Autodesk Fusion 360 part; units mm, degrees
note: some values were not read from the file. Set by a fixed rule: which sketch regions a step uses.
(part 2 of 15)
  line L768 (243.501, -127.288) -> (243.645, -127.172)
  line L769 (233.618, -130.511) -> (233.477, -130.391)
  line L770 (245.044, -127.604) -> (245.097, -127.782)
  line L771 (245.116, -127.966) -> (245.115, -127.993)
  line L772 (244.675, -128.769) -> (244.509, -128.852)
  line L773 (243.482, -128.626) -> (243.367, -128.481)
  line L774 (101.127, -129.506) -> (101.145, -129.691)
  line L775 (244.509, -128.852) -> (244.331, -128.902)
  line L776 (99.2447, -129.677) -> (99.2654, -129.493)
  line L777 (99.8143, -130.561) -> (99.6524, -130.471)
  line L778 (100.201, -128.741) -> (100.386, -128.76)
  line L779 (233.982, -128.798) -> (234.167, -128.781)
  line L780 (99.6524, -130.471) -> (99.5112, -130.351)
  line L781 (244.357, -127.036) -> (244.534, -127.091)
  line L782 (99.6744, -128.896) -> (99.8387, -128.81)
  line L783 (245.097, -127.782) -> (245.116, -127.966)
  line L784 (243.382, -127.43) -> (243.501, -127.288)
  line L785 (100.36, -130.626) -> (100.175, -130.64)
  line L786 (243.236, -127.769) -> (243.292, -127.592)
  line L787 (243.292, -127.592) -> (243.382, -127.43)
  line L788 (244.172, -127.017) -> (244.357, -127.036)
  line L789 (99.4108, -129.154) -> (99.5299, -129.012)
  line L790 (244.942, -128.514) -> (244.821, -128.654)
  line L791 (245.092, -128.177) -> (245.033, -128.353)
  line L792 (99.3214, -129.316) -> (99.4108, -129.154)
  line L793 (245.115, -127.993) -> (245.092, -128.177)
  line L794 (99.5299, -129.012) -> (99.6744, -128.896)
  line L795 (243.81, -127.086) -> (243.988, -127.033)
  line L796 (243.988, -127.033) -> (244.172, -127.017)
  line L797 (233.225, -129.902) -> (233.21, -129.717)
  line L798 (244.84, -127.297) -> (244.957, -127.441)
  line L799 (100.017, -128.758) -> (100.201, -128.741)
  line L800 (99.8387, -128.81) -> (100.017, -128.758)
  line L801 (243.216, -127.953) -> (243.236, -127.769)
  line L802 (243.623, -128.747) -> (243.482, -128.626)
  line L803 (101.073, -129.329) -> (101.127, -129.506)
  line L804 (234.14, -130.681) -> (233.956, -130.659)
  line L805 (243.962, -128.894) -> (243.785, -128.837)
  line L806 (233.956, -130.659) -> (233.78, -130.601)
  line L807 (233.78, -130.601) -> (233.618, -130.511)
  line L808 (99.2654, -129.493) -> (99.3214, -129.316)
  line L809 (99.9906, -130.619) -> (99.8143, -130.561)
  line L810 (99.2602, -129.862) -> (99.2447, -129.677)
  line L811 (243.785, -128.837) -> (243.623, -128.747)
  line L812 (245.033, -128.353) -> (244.942, -128.514)
  line L813 (99.5112, -130.351) -> (99.3961, -130.205)
  line L814 (91.1154, -128.137) -> (91.0568, -128.313)
  line L815 (91.0568, -128.313) -> (90.9653, -128.474)
  line L816 (244.146, -128.916) -> (243.962, -128.894)
  line L817 (234.167, -128.781) -> (234.351, -128.8)
  line L818 (244.821, -128.654) -> (244.675, -128.769)
  line L819 (99.3961, -130.205) -> (99.3113, -130.04)
  line L820 (99.3113, -130.04) -> (99.2602, -129.862)
  line L821 (233.231, -129.533) -> (233.287, -129.357)
  line L822 (100.538, -130.576) -> (100.36, -130.626)
  line L823 (244.957, -127.441) -> (245.044, -127.604)
  line L824 (89.2391, -127.913) -> (89.2597, -127.729)
  line L825 (258.114, -121.378) -> (258.378, -121.48)
  line L826 (89.4051, -127.39) -> (89.5243, -127.248)
  line L827 (91.0673, -127.564) -> (91.1209, -127.742)
  line L828 (243.231, -128.138) -> (243.216, -127.953)
  line L829 (90.7202, -127.139) -> (90.8631, -127.257)
  line L830 (91.1209, -127.742) -> (91.139, -127.926)
  line L831 (258.378, -121.48) -> (258.624, -121.618)
  line L832 (90.698, -128.729) -> (90.5325, -128.812)
  line L833 (259.215, -122.218) -> (259.349, -122.466)
  line L834 (259.349, -122.466) -> (259.447, -122.731)
  line L835 (259.506, -123.008) -> (259.526, -123.289)
  line L836 (89.6468, -128.707) -> (89.5056, -128.586)
  line L837 (89.3158, -127.552) -> (89.4051, -127.39)
  line L838 (259.526, -123.289) -> (259.522, -123.415)
  line L839 (90.5325, -128.812) -> (90.3539, -128.862)
  line L840 (89.8331, -127.046) -> (90.011, -126.993)
  line L841 (90.8441, -128.614) -> (90.698, -128.729)
  line L842 (91.1386, -127.953) -> (91.1154, -128.137)
  line L843 (90.3539, -128.862) -> (90.1691, -128.876)
  line L844 (90.5571, -127.051) -> (90.7202, -127.139)
  line L845 (90.9802, -127.401) -> (91.0673, -127.564)
  line L846 (89.3904, -128.441) -> (89.3057, -128.276)
  line L847 (89.8086, -128.797) -> (89.6468, -128.707)
  line L848 (89.2597, -127.729) -> (89.3158, -127.552)
  line L849 (257.839, -121.314) -> (258.114, -121.378)
  line L850 (258.624, -121.618) -> (258.849, -121.789)
  line L851 (258.849, -121.789) -> (259.047, -121.99)
  line L852 (259.447, -122.731) -> (259.506, -123.008)
  line L853 (244.331, -128.902) -> (244.146, -128.916)
  line L854 (243.645, -127.172) -> (243.81, -127.086)
  line L855 (89.6688, -127.131) -> (89.8331, -127.046)
  line L856 (90.011, -126.993) -> (90.1956, -126.976)
  line L857 (90.1691, -128.876) -> (89.985, -128.854)
  line L858 (89.2546, -128.098) -> (89.2391, -127.913)
  line L859 (91.139, -127.926) -> (91.1386, -127.953)
  line L860 (90.38, -126.996) -> (90.5571, -127.051)
  line L861 (259.047, -121.99) -> (259.215, -122.218)
  line L862 (89.985, -128.854) -> (89.8086, -128.797)
  line L863 (90.1956, -126.976) -> (90.38, -126.996)
  line L864 (243.282, -128.316) -> (243.231, -128.138)
  line L865 (89.5056, -128.586) -> (89.3904, -128.441)
  line L866 (255.73, -122.409) -> (255.872, -122.165)
  line L867 (256.251, -121.748) -> (256.481, -121.584)
  line L868 (89.5243, -127.248) -> (89.6688, -127.131)
  line L869 (89.3057, -128.276) -> (89.2546, -128.098)
  line L870 (90.8631, -127.257) -> (90.9802, -127.401)
  line L871 (90.9653, -128.474) -> (90.8441, -128.614)
  line L872 (257.993, -125.234) -> (257.715, -125.28)
  line L873 (257.715, -125.28) -> (257.432, -125.287)
  line L874 (255.538, -123.509) -> (255.527, -123.227)
  line L875 (56.6309, -103.238) -> (56.4848, -103.352)
  line L876 (298.503, -101.671) -> (298.556, -101.849)
  line L877 (55.4336, -103.33) -> (55.2924, -103.21)
  line L878 (55.5955, -103.42) -> (55.4336, -103.33)
  line L879 (55.0466, -102.352) -> (55.1026, -102.176)
  line L880 (55.3111, -101.871) -> (55.4556, -101.755)
  line L881 (298.556, -101.849) -> (298.574, -102.033)
  line L882 (298.416, -101.508) -> (298.503, -101.671)
  line L883 (298.299, -101.364) -> (298.416, -101.508)
  line L884 (298.551, -102.244) -> (298.492, -102.42)
  line L885 (55.9559, -103.5) -> (55.7718, -103.478)
  line L886 (55.1026, -102.176) -> (55.1919, -102.013)
  line L887 (55.0925, -102.9) -> (55.0414, -102.721)
  line L888 (55.7978, -101.617) -> (55.9824, -101.6)
  line L889 (298.574, -102.06) -> (298.551, -102.244)
  line L890 (56.4848, -103.352) -> (56.3193, -103.436)
  line L891 (55.2924, -103.21) -> (55.1773, -103.064)
  line L892 (55.9824, -101.6) -> (56.1668, -101.619)
  line L893 (55.0414, -102.721) -> (55.0259, -102.537)
  line L894 (297.993, -101.158) -> (298.156, -101.246)
  line L895 (55.4556, -101.755) -> (55.6199, -101.669)
  line L896 (297.815, -101.103) -> (297.993, -101.158)
  line L897 (298.574, -102.033) -> (298.574, -102.06)
  line L898 (55.0259, -102.537) -> (55.0466, -102.352)
  line L899 (55.1919, -102.013) -> (55.3111, -101.871)
  line L900 (59.8286, -105.068) -> (59.6095, -104.89)
  line L901 (269.323, -104.381) -> (269.299, -104.565)
  line L902 (269.149, -104.902) -> (269.028, -105.042)
  line L903 (269.028, -105.042) -> (268.882, -105.156)
  line L904 (59.0765, -102.814) -> (59.1826, -102.552)
  line L905 (268.904, -103.567) -> (269.047, -103.685)
  line L906 (268.564, -103.424) -> (268.741, -103.478)
  line L907 (58.9796, -103.369) -> (59.0084, -103.088)
  line L908 (66.9311, -104.341) -> (66.9078, -104.525)
  line L909 (66.9078, -104.525) -> (66.8493, -104.7)
  line L910 (267.49, -104.704) -> (267.439, -104.526)
  line L911 (267.5, -103.98) -> (267.589, -103.817)
  line L912 (268.195, -103.421) -> (268.38, -103.404)
  line L913 (66.3496, -103.438) -> (66.5127, -103.527)
  line L914 (268.017, -103.473) -> (268.195, -103.421)
  line L915 (267.831, -105.134) -> (267.69, -105.014)
  line L916 (65.1829, -104.829) -> (65.0981, -104.664)
  line L917 (294.542, -102.358) -> (294.602, -102.634)
  line L918 (65.1083, -103.94) -> (65.1976, -103.777)
  line L919 (66.9133, -104.13) -> (66.9314, -104.314)
  line L920 (65.7774, -105.242) -> (65.6011, -105.185)
  line L921 (66.7727, -103.788) -> (66.8598, -103.952)
  line L922 (59.7038, -101.891) -> (59.9336, -101.727)
  line L923 (66.9314, -104.314) -> (66.9311, -104.341)
  line L924 (66.8493, -104.7) -> (66.7577, -104.862)
  line L925 (66.6555, -103.645) -> (66.7727, -103.788)
  line L926 (268.538, -105.29) -> (268.353, -105.304)
  line L927 (267.423, -104.341) -> (267.444, -104.157)
  line L928 (59.4994, -102.086) -> (59.7038, -101.891)
  line L929 (267.993, -105.225) -> (267.831, -105.134)
  line L930 (267.589, -103.817) -> (267.708, -103.675)
  line L931 (268.353, -105.304) -> (268.169, -105.282)
  line L932 (66.8598, -103.952) -> (66.9133, -104.13)
  line L933 (66.7577, -104.862) -> (66.6366, -105.002)
  line L934 (267.575, -104.869) -> (267.49, -104.704)
  line L935 (267.439, -104.526) -> (267.423, -104.341)
  line L936 (268.169, -105.282) -> (267.993, -105.225)
  line L937 (267.853, -103.559) -> (268.017, -103.473)
  line L938 (66.1725, -103.384) -> (66.3496, -103.438)
  line L939 (267.444, -104.157) -> (267.5, -103.98)
  line L940 (267.708, -103.675) -> (267.853, -103.559)
  line L941 (268.882, -105.156) -> (268.717, -105.24)
  line L942 (268.38, -103.404) -> (268.564, -103.424)
  line L943 (66.5127, -103.527) -> (66.6555, -103.645)
  line L944 (268.717, -105.24) -> (268.538, -105.29)
  line L945 (267.69, -105.014) -> (267.575, -104.869)
  line L946 (269.251, -103.992) -> (269.305, -104.17)
  line L947 (60.7279, -101.448) -> (61.01, -101.432)
  line L948 (60.1843, -101.596) -> (60.4509, -101.503)
  line L949 (269.241, -104.741) -> (269.149, -104.902)
  line L950 (59.0084, -103.088) -> (59.0765, -102.814)
  line L951 (59.9336, -101.727) -> (60.1843, -101.596)
  line L952 (269.299, -104.565) -> (269.241, -104.741)
  line L953 (269.323, -104.354) -> (269.323, -104.381)
  line L954 (61.01, -101.432) -> (61.2915, -101.457)
  line L955 (59.2571, -104.45) -> (59.1309, -104.197)
  line L956 (269.305, -104.17) -> (269.323, -104.354)
  line L957 (269.164, -103.828) -> (269.251, -103.992)
  line L958 (59.0414, -103.929) -> (58.9907, -103.651)
  line L959 (60.4509, -101.503) -> (60.7279, -101.448)
  line L960 (268.741, -103.478) -> (268.904, -103.567)
  line L961 (269.047, -103.685) -> (269.164, -103.828)
  line L962 (59.4178, -104.682) -> (59.2571, -104.45)
  line L963 (59.3245, -102.308) -> (59.4994, -102.086)
  line L964 (59.1826, -102.552) -> (59.3245, -102.308)
  line L965 (59.6095, -104.89) -> (59.4178, -104.682)
  line L966 (109.335, -72.8722) -> (109.454, -72.7302)
  line L967 (278.888, -103.392) -> (278.722, -103.476)
  line L968 (56.3439, -101.674) -> (56.507, -101.762)
  line L969 (278.359, -103.54) -> (278.175, -103.518)
  line L970 (55.1773, -103.064) -> (55.0925, -102.9)
  line L971 (277.495, -102.94) -> (277.444, -102.761)
  line L972 (278.201, -101.657) -> (278.385, -101.64)
  line L973 (277.444, -102.761) -> (277.429, -102.577)
  line L974 (278.175, -103.518) -> (277.998, -103.46)
  line L975 (278.385, -101.64) -> (278.57, -101.659)
  line L976 (278.722, -103.476) -> (278.544, -103.525)
  line L977 (298.156, -101.246) -> (298.299, -101.364)
  line L978 (56.3193, -103.436) -> (56.1408, -103.485)
  line L979 (74.2602, -103.232) -> (74.3495, -103.07)
  line L980 (279.053, -101.92) -> (279.17, -102.064)
  line L981 (279.155, -103.138) -> (279.034, -103.278)
  line L982 (74.753, -104.477) -> (74.5912, -104.387)
  line L983 (56.9077, -102.365) -> (56.9258, -102.55)
  line L984 (277.859, -101.795) -> (278.023, -101.709)
  line L985 (277.695, -103.25) -> (277.58, -103.105)
  line L986 (277.429, -102.577) -> (277.449, -102.392)
  line L987 (277.714, -101.911) -> (277.859, -101.795)
  line L988 (56.1668, -101.619) -> (56.3439, -101.674)
  line L989 (277.595, -102.053) -> (277.714, -101.911)
  line L990 (74.3495, -103.07) -> (74.4687, -102.928)
  line L991 (74.1989, -103.778) -> (74.1834, -103.593)
  line L992 (277.506, -102.216) -> (277.595, -102.053)
  line L993 (74.2501, -103.956) -> (74.1989, -103.778)
  line L994 (279.257, -102.228) -> (279.311, -102.405)
  line L995 (56.7671, -102.024) -> (56.8541, -102.188)
  line L996 (277.449, -102.392) -> (277.506, -102.216)
  line L997 (279.328, -102.616) -> (279.305, -102.8)
  line L998 (279.329, -102.59) -> (279.328, -102.616)
  line L999 (74.9293, -104.534) -> (74.753, -104.477)
  line L1000 (279.034, -103.278) -> (278.888, -103.392)
  line L1001 (56.9254, -102.576) -> (56.9022, -102.76)
  line L1002 (56.6499, -101.88) -> (56.7671, -102.024)
  line L1003 (56.9022, -102.76) -> (56.8437, -102.936)
  line L1004 (279.305, -102.8) -> (279.247, -102.976)
  line L1005 (56.9258, -102.55) -> (56.9254, -102.576)
  line L1006 (278.57, -101.659) -> (278.747, -101.714)
  line L1007 (56.8437, -102.936) -> (56.7521, -103.097)
  line L1008 (56.7521, -103.097) -> (56.6309, -103.238)
  line L1009 (56.8541, -102.188) -> (56.9077, -102.365)
  line L1010 (278.023, -101.709) -> (278.201, -101.657)
  line L1011 (277.998, -103.46) -> (277.837, -103.37)
  line L1012 (278.544, -103.525) -> (278.359, -103.54)
  line L1013 (56.507, -101.762) -> (56.6499, -101.88)
  line L1014 (277.837, -103.37) -> (277.695, -103.25)
  line L1015 (75.4769, -104.492) -> (75.2983, -104.542)
  line L1016 (277.58, -103.105) -> (277.495, -102.94)
  line L1017 (74.2041, -103.409) -> (74.2602, -103.232)
  line L1018 (74.4687, -102.928) -> (74.6132, -102.812)
  line L1019 (279.247, -102.976) -> (279.155, -103.138)
  line L1020 (278.747, -101.714) -> (278.91, -101.802)
  line L1021 (74.45, -104.266) -> (74.3348, -104.121)
  line L1022 (30.5232, -111.407) -> (30.7847, -111.468)
  line L1023 (112.793, -114.541) -> (112.811, -114.725)
  line L1024 (112.652, -114.199) -> (112.739, -114.363)
  line L1025 (112.516, -115.413) -> (112.37, -115.527)
  line L1026 (111.318, -115.505) -> (111.177, -115.385)
  line L1027 (112.204, -115.611) -> (112.026, -115.661)
  line L1028 (111.177, -115.385) -> (111.062, -115.24)
  line L1029 (112.787, -114.936) -> (112.728, -115.111)
  line L1030 (111.062, -115.24) -> (110.977, -115.075)
  line L1031 (111.34, -113.93) -> (111.505, -113.844)
  line L1032 (112.637, -115.273) -> (112.516, -115.413)
  line L1033 (111.841, -115.675) -> (111.657, -115.653)
  line L1034 (111.196, -114.046) -> (111.34, -113.93)
  line L1035 (32.0506, -112.754) -> (32.107, -113.016)
  line L1036 (28.9254, -114.669) -> (28.7432, -114.472)
  line L1037 (29.6106, -115.082) -> (29.3634, -114.977)
  line L1038 (31.4825, -111.859) -> (31.6708, -112.05)
  line L1039 (111.077, -114.188) -> (111.196, -114.046)
  line L1040 (31.9052, -114.173) -> (31.7631, -114.401)
  line L1041 (31.5904, -114.606) -> (31.3905, -114.785)
  line L1042 (32.0137, -113.928) -> (31.9052, -114.173)
  line L1043 (31.7631, -114.401) -> (31.5904, -114.606)
  line L1044 (31.1674, -114.934) -> (30.9254, -115.051)
  line L1045 (31.2691, -111.696) -> (31.4825, -111.859)
  line L1046 (29.3634, -114.977) -> (29.1335, -114.838)
  line L1047 (30.1365, -115.182) -> (29.87, -115.15)
  line L1048 (28.3857, -113.757) -> (28.3375, -113.492)
  line L1049 (31.3905, -114.785) -> (31.1674, -114.934)
  line L1050 (28.4706, -114.011) -> (28.3857, -113.757)
  line L1051 (31.9577, -112.502) -> (32.0506, -112.754)
  line L1052 (30.7847, -111.468) -> (31.035, -111.565)
  line L1053 (31.035, -111.565) -> (31.2691, -111.696)
  line L1054 (30.4048, -115.176) -> (30.1365, -115.182)
  line L1055 (29.87, -115.15) -> (29.6106, -115.082)
  line L1056 (31.6708, -112.05) -> (31.8302, -112.266)
  line L1057 (28.5906, -114.251) -> (28.4706, -114.011)
  line L1058 (30.9254, -115.051) -> (30.6695, -115.132)
  line L1059 (28.3375, -113.492) -> (28.3269, -113.224)
  line L1060 (32.107, -113.016) -> (32.126, -113.284)
  line L1061 (31.8302, -112.266) -> (31.9577, -112.502)
  line L1062 (30.6695, -115.132) -> (30.4048, -115.176)
  line L1063 (32.126, -113.284) -> (32.1223, -113.403)
  line L1064 (28.7432, -114.472) -> (28.5906, -114.251)
  line L1065 (116.489, -117.572) -> (116.216, -117.499)
  line L1066 (114.893, -115.263) -> (114.961, -114.989)
  line L1067 (115.209, -114.483) -> (115.384, -114.261)
  line L1068 (116.216, -117.499) -> (115.955, -117.389)
  line L1069 (114.864, -115.544) -> (114.893, -115.263)
  line L1070 (212.856, -115.654) -> (213.019, -115.742)
  line L1071 (211.554, -116.701) -> (211.538, -116.516)
  line L1072 (213.438, -116.556) -> (213.415, -116.74)
  line L1073 (116.895, -113.607) -> (117.176, -113.632)
  line L1074 (212.679, -115.599) -> (212.856, -115.654)
  line L1075 (117.6, -117.467) -> (117.33, -117.552)
  line L1076 (117.33, -117.552) -> (117.052, -117.598)
  line L1077 (115.142, -116.625) -> (115.016, -116.373)
  line L1078 (213.438, -116.529) -> (213.438, -116.556)
  line L1079 (211.538, -116.516) -> (211.559, -116.332)
  line L1080 (122.234, -115.614) -> (122.397, -115.702)
  line L1081 (116.613, -113.623) -> (116.895, -113.607)
  line L1082 (115.384, -114.261) -> (115.589, -114.066)
  line L1083 (122.397, -115.702) -> (122.54, -115.82)
  line L1084 (114.961, -114.989) -> (115.067, -114.727)
  line L1085 (211.704, -115.993) -> (211.824, -115.851)
  line L1086 (215.695, -114.767) -> (215.837, -114.523)
  line L1087 (115.713, -117.244) -> (115.494, -117.065)
  line L1088 (213.143, -117.217) -> (212.997, -117.332)
  line L1089 (122.057, -115.559) -> (122.234, -115.614)
  line L1090 (213.42, -116.345) -> (213.438, -116.529)
  line L1091 (117.052, -117.598) -> (116.769, -117.605)
  line L1092 (122.54, -115.82) -> (122.658, -115.964)
  line L1093 (213.367, -116.167) -> (213.42, -116.345)
  line L1094 (213.28, -116.004) -> (213.367, -116.167)
  line L1095 (213.415, -116.74) -> (213.356, -116.916)
  line L1096 (215.837, -114.523) -> (216.012, -114.301)
  line L1097 (115.589, -114.066) -> (115.818, -113.902)
  line L1098 (116.336, -113.678) -> (116.613, -113.623)
  line L1099 (115.303, -116.858) -> (115.142, -116.625)
  line L1100 (211.824, -115.851) -> (211.968, -115.735)
  line L1101 (212.132, -115.649) -> (212.31, -115.596)
  line L1102 (115.818, -113.902) -> (116.069, -113.772)
  line L1103 (216.446, -113.942) -> (216.697, -113.812)
  line L1104 (116.069, -113.772) -> (116.336, -113.678)
  line L1105 (115.494, -117.065) -> (115.303, -116.858)
  line L1106 (212.997, -117.332) -> (212.832, -117.415)
  line L1107 (114.875, -115.827) -> (114.864, -115.544)
  line L1108 (213.265, -117.077) -> (213.143, -117.217)
  line L1109 (215.492, -115.584) -> (215.521, -115.303)
  line L1110 (115.955, -117.389) -> (115.713, -117.244)
  line L1111 (114.926, -116.105) -> (114.875, -115.827)
  line L1112 (213.162, -115.86) -> (213.28, -116.004)
  line L1113 (212.495, -115.579) -> (212.679, -115.599)
  line L1114 (115.067, -114.727) -> (115.209, -114.483)
  line L1115 (213.019, -115.742) -> (213.162, -115.86)
  line L1116 (115.016, -116.373) -> (114.926, -116.105)
  line L1117 (116.769, -117.605) -> (116.489, -117.572)
  line L1118 (-10.9606, -114.234) -> (-10.7834, -114.289)
  line L1119 (122.521, -117.177) -> (122.375, -117.291)
  line L1120 (121.846, -117.439) -> (121.662, -117.417)
  line L1121 (122.031, -117.425) -> (121.846, -117.439)
  line L1122 (211.946, -117.31) -> (211.805, -117.189)
  line L1123 (211.559, -116.332) -> (211.615, -116.155)
  line L1124 (-10.2197, -114.98) -> (-10.2016, -115.165)
  line L1125 (212.284, -117.457) -> (212.108, -117.4)
  line L1126 (-10.9866, -116.1) -> (-11.1715, -116.114)
  line L1127 (121.486, -117.36) -> (121.324, -117.269)
  line L1128 (122.745, -116.127) -> (122.798, -116.305)
  line L1129 (-11.8163, -114.486) -> (-11.6718, -114.37)
  line L1130 (122.793, -116.7) -> (122.734, -116.876)
  line L1131 (-11.1449, -114.215) -> (-10.9606, -114.234)
  line L1132 (-12.1015, -115.151) -> (-12.0808, -114.967)
  line L1133 (222.685, -113.835) -> (222.862, -113.889)
  line L1134 (-10.808, -116.05) -> (-10.9866, -116.1)
  line L1135 (121.082, -115.953) -> (121.202, -115.811)
  line L1136 (-10.6425, -115.967) -> (-10.808, -116.05)
  line L1137 (212.653, -117.465) -> (212.468, -117.479)
  line L1138 (-10.7834, -114.289) -> (-10.6203, -114.377)
  line L1139 (121.873, -115.539) -> (122.057, -115.559)
  line L1140 (-10.4775, -114.495) -> (-10.3603, -114.639)
  line L1141 (121.346, -115.694) -> (121.51, -115.609)
  line L1142 (121.51, -115.609) -> (121.688, -115.556)
  line L1143 (122.375, -117.291) -> (122.21, -117.375)
  line L1144 (121.688, -115.556) -> (121.873, -115.539)
  line L1145 (-10.3753, -115.712) -> (-10.4964, -115.853)
  line L1146 (211.605, -116.879) -> (211.554, -116.701)
  line L1147 (212.468, -117.479) -> (212.284, -117.457)
  line L1148 (212.31, -115.596) -> (212.495, -115.579)
  line L1149 (121.662, -117.417) -> (121.486, -117.36)
  line L1150 (120.983, -116.839) -> (120.932, -116.661)
  line L1151 (-11.6718, -114.37) -> (-11.5075, -114.284)
  line L1152 (-12.086, -115.336) -> (-12.1015, -115.151)
  line L1153 (-11.3296, -114.231) -> (-11.1449, -114.215)
  line L1154 (-11.5075, -114.284) -> (-11.3296, -114.231)
  line L1155 (212.108, -117.4) -> (211.946, -117.31)
  line L1156 (212.832, -117.415) -> (212.653, -117.465)
  line L1157 (211.805, -117.189) -> (211.69, -117.044)
  line L1158 (122.21, -117.375) -> (122.031, -117.425)
  line L1159 (122.798, -116.305) -> (122.816, -116.489)
  line L1160 (120.916, -116.476) -> (120.937, -116.292)
  line L1161 (-10.2837, -115.551) -> (-10.3753, -115.712)
  line L1162 (-11.1715, -116.114) -> (-11.3556, -116.092)
  line L1163 (121.183, -117.149) -> (121.068, -117.004)
  line L1164 (121.068, -117.004) -> (120.983, -116.839)
  line L1165 (122.816, -116.489) -> (122.816, -116.516)
  line L1166 (-10.6203, -114.377) -> (-10.4775, -114.495)
  line L1167 (121.202, -115.811) -> (121.346, -115.694)
  line L1168 (122.816, -116.516) -> (122.793, -116.7)
  line L1169 (121.324, -117.269) -> (121.183, -117.149)
  line L1170 (120.932, -116.661) -> (120.916, -116.476)
  line L1171 (211.69, -117.044) -> (211.605, -116.879)
  line L1172 (120.937, -116.292) -> (120.993, -116.115)
  line L1173 (122.643, -117.037) -> (122.521, -117.177)
  line L1174 (-10.2016, -115.165) -> (-10.2019, -115.191)
  line L1175 (-10.2019, -115.191) -> (-10.2252, -115.375)
  line L1176 (122.658, -115.964) -> (122.745, -116.127)
  line L1177 (213.356, -116.916) -> (213.265, -117.077)
  line L1178 (122.734, -116.876) -> (122.643, -117.037)
  line L1179 (120.993, -116.115) -> (121.082, -115.953)
  line L1180 (211.615, -116.155) -> (211.704, -115.993)
  line L1181 (211.968, -115.735) -> (212.132, -115.649)
  line L1182 (221.695, -115.28) -> (221.611, -115.115)
  line L1183 (-10.2252, -115.375) -> (-10.2837, -115.551)
  line L1184 (222.316, -113.832) -> (222.501, -113.815)
  line L1185 (-12.0808, -114.967) -> (-12.0248, -114.79)
  line L1186 (223.444, -114.765) -> (223.444, -114.792)
  line L1187 (222.29, -115.693) -> (222.114, -115.636)
  line L1188 (223.362, -115.152) -> (223.27, -115.313)
  line L1189 (222.474, -115.715) -> (222.29, -115.693)
  line L1190 (222.501, -113.815) -> (222.685, -113.835)
  line L1191 (221.544, -114.752) -> (221.565, -114.568)
  line L1192 (-11.835, -115.824) -> (-11.9501, -115.679)
  line L1193 (223.285, -114.239) -> (223.372, -114.403)
  line L1194 (-10.3603, -114.639) -> (-10.2733, -114.803)
  line L1195 (223.025, -113.978) -> (223.168, -114.096)
  line L1196 (112.026, -115.661) -> (111.841, -115.675)
  line L1197 (-12.0248, -114.79) -> (-11.9354, -114.628)
  line L1198 (223.149, -115.453) -> (223.003, -115.567)
  line L1199 (112.052, -113.795) -> (112.229, -113.849)
  line L1200 (223.42, -114.976) -> (223.362, -115.152)
  line L1201 (111.48, -115.596) -> (111.318, -115.505)
  line L1202 (222.138, -113.884) -> (222.316, -113.832)
  line L1203 (223.444, -114.792) -> (223.42, -114.976)
  line L1204 (110.911, -114.712) -> (110.931, -114.528)
  line L1205 (221.829, -114.086) -> (221.974, -113.97)
  line L1206 (112.37, -115.527) -> (112.204, -115.611)
  line L1207 (112.535, -114.056) -> (112.652, -114.199)
  line L1208 (221.621, -114.391) -> (221.71, -114.228)
  line L1209 (112.739, -114.363) -> (112.793, -114.541)
  line L1210 (-11.9501, -115.679) -> (-12.0349, -115.514)
  line L1211 (221.974, -113.97) -> (222.138, -113.884)
  line L1212 (112.229, -113.849) -> (112.392, -113.938)
  line L1213 (221.952, -115.545) -> (221.811, -115.425)
  line L1214 (223.27, -115.313) -> (223.149, -115.453)
  line L1215 (222.659, -115.701) -> (222.474, -115.715)
  line L1216 (112.392, -113.938) -> (112.535, -114.056)
  line L1217 (111.657, -115.653) -> (111.48, -115.596)
  line L1218 (223.003, -115.567) -> (222.837, -115.651)
  line L1219 (223.168, -114.096) -> (223.285, -114.239)
  line L1220 (112.81, -114.752) -> (112.787, -114.936)
  line L1221 (222.837, -115.651) -> (222.659, -115.701)
  line L1222 (-11.3556, -116.092) -> (-11.5319, -116.035)
  line L1223 (223.372, -114.403) -> (223.426, -114.581)
  line L1224 (221.565, -114.568) -> (221.621, -114.391)
  line L1225 (112.728, -115.111) -> (112.637, -115.273)
  line L1226 (111.683, -113.792) -> (111.867, -113.775)
  line L1227 (221.71, -114.228) -> (221.829, -114.086)
  line L1228 (-10.2733, -114.803) -> (-10.2197, -114.98)
  line L1229 (221.611, -115.115) -> (221.56, -114.937)
  line L1230 (221.56, -114.937) -> (221.544, -114.752)
  line L1231 (112.811, -114.725) -> (112.81, -114.752)
  line L1232 (110.977, -115.075) -> (110.926, -114.897)
  line L1233 (110.926, -114.897) -> (110.911, -114.712)
  line L1234 (110.987, -114.351) -> (111.077, -114.188)
  line L1235 (111.505, -113.844) -> (111.683, -113.792)
  line L1236 (-11.6938, -115.945) -> (-11.835, -115.824)
  line L1237 (-12.0349, -115.514) -> (-12.086, -115.336)
  line L1238 (110.931, -114.528) -> (110.987, -114.351)
  line L1239 (222.114, -115.636) -> (221.952, -115.545)
  line L1240 (-11.9354, -114.628) -> (-11.8163, -114.486)
  line L1241 (-11.5319, -116.035) -> (-11.6938, -115.945)
  line L1242 (223.426, -114.581) -> (223.444, -114.765)
  line L1243 (221.811, -115.425) -> (221.695, -115.28)
  line L1244 (222.862, -113.889) -> (223.025, -113.978)
  line L1245 (-10.4964, -115.853) -> (-10.6425, -115.967)
  line L1246 (111.867, -113.775) -> (112.052, -113.795)
  line L1247 (294.31, -101.844) -> (294.444, -102.093)
  line L1248 (65.0522, -104.117) -> (65.1083, -103.94)
  line L1249 (65.0981, -104.664) -> (65.047, -104.486)
  line L1250 (294.602, -102.634) -> (294.622, -102.916)
  line L1251 (65.8034, -103.381) -> (65.9881, -103.364)
  line L1252 (293.944, -101.415) -> (294.142, -101.617)
  line L1253 (65.9615, -105.264) -> (65.7774, -105.242)
  line L1254 (66.6366, -105.002) -> (66.4905, -105.116)
  line L1255 (65.0315, -104.301) -> (65.0522, -104.117)
  line L1256 (293.473, -101.106) -> (293.72, -101.244)
  line L1257 (65.2981, -104.974) -> (65.1829, -104.829)
  line L1258 (66.1464, -105.25) -> (65.9615, -105.264)
  line L1259 (66.325, -105.2) -> (66.1464, -105.25)
  line L1260 (294.142, -101.617) -> (294.31, -101.844)
  line L1261 (294.444, -102.093) -> (294.542, -102.358)
  line L1262 (290.684, -103.413) -> (290.634, -103.135)
  line L1263 (290.9, -103.934) -> (290.774, -103.681)
  line L1264 (294.618, -103.041) -> (294.58, -103.321)
  line L1265 (294.24, -104.091) -> (294.058, -104.307)
  line L1266 (291.347, -101.375) -> (291.577, -101.21)
  line L1267 (290.967, -101.791) -> (291.142, -101.57)
  line L1268 (293.089, -104.86) -> (292.81, -104.907)
  line L1269 (291.061, -104.166) -> (290.9, -103.934)
  line L1270 (294.58, -103.321) -> (294.503, -103.593)
  line L1271 (291.827, -101.08) -> (292.094, -100.986)
  line L1272 (294.058, -104.307) -> (293.847, -104.496)
  line L1273 (291.253, -104.374) -> (291.061, -104.166)
  line L1274 (292.81, -104.907) -> (292.527, -104.913)
  line L1275 (291.142, -101.57) -> (291.347, -101.375)
  line L1276 (291.974, -104.808) -> (291.714, -104.698)
  line L1277 (290.623, -102.853) -> (290.651, -102.572)
  line L1278 (293.613, -104.653) -> (293.358, -104.775)
  line L1279 (290.774, -103.681) -> (290.684, -103.413)
  line L1280 (291.472, -104.552) -> (291.253, -104.374)
  line L1281 (290.826, -102.036) -> (290.967, -101.791)
  line L1282 (290.72, -102.298) -> (290.826, -102.036)
  line L1283 (292.094, -100.986) -> (292.371, -100.931)
  line L1284 (293.847, -104.496) -> (293.613, -104.653)
  line L1285 (294.389, -103.851) -> (294.24, -104.091)
  line L1286 (291.714, -104.698) -> (291.472, -104.552)
  line L1287 (291.577, -101.21) -> (291.827, -101.08)
  line L1288 (292.527, -104.913) -> (292.247, -104.88)
  line L1289 (290.634, -103.135) -> (290.623, -102.853)
  line L1290 (292.247, -104.88) -> (291.974, -104.808)
  line L1291 (294.503, -103.593) -> (294.389, -103.851)
  line L1292 (290.651, -102.572) -> (290.72, -102.298)
  line L1293 (293.358, -104.775) -> (293.089, -104.86)
  line L1294 (294.622, -102.916) -> (294.618, -103.041)
  line L1295 (293.21, -101.004) -> (293.473, -101.106)
  line L1296 (66.4905, -105.116) -> (66.325, -105.2)
  line L1297 (293.72, -101.244) -> (293.944, -101.415)
  line L1298 (65.9881, -103.364) -> (66.1725, -103.384)
  line L1299 (65.3168, -103.635) -> (65.4613, -103.519)
  line L1300 (65.047, -104.486) -> (65.0315, -104.301)
  line L1301 (65.1976, -103.777) -> (65.3168, -103.635)
  line L1302 (65.4393, -105.094) -> (65.2981, -104.974)
  line L1303 (65.6011, -105.185) -> (65.4393, -105.094)
  line L1304 (65.4613, -103.519) -> (65.6256, -103.433)
  line L1305 (65.6256, -103.433) -> (65.8034, -103.381)
  line L1306 (292.935, -100.94) -> (293.21, -101.004)
  line L1307 (17.0862, -99.0351) -> (17.035, -98.8569)
  line L1308 (-1.9892, -95.4764) -> (-1.7427, -95.6145)
  line L1309 (-4.6368, -96.4062) -> (-4.4949, -96.1619)
  line L1310 (-0.8447, -97.4117) -> (-0.8823, -97.6917)
  line L1311 (17.2861, -99.3453) -> (17.1709, -99.2)
  line L1312 (17.0963, -98.3111) -> (17.1856, -98.1487)
  line L1313 (18.8958, -98.8959) -> (18.8373, -99.0718)
  line L1314 (17.0195, -98.6721) -> (17.0402, -98.4879)
  line L1315 (17.035, -98.8569) -> (17.0195, -98.6721)
  line L1316 (17.6136, -97.8046) -> (17.7914, -97.7522)
  line L1317 (-4.7429, -96.668) -> (-4.6368, -96.4062)
  line L1318 (17.3048, -98.0066) -> (17.4493, -97.8905)
  line L1319 (-1.8498, -99.0233) -> (-2.1045, -99.1456)
  line L1320 (18.4785, -99.4875) -> (18.313, -99.5711)
  line L1321 (-4.2099, -98.744) -> (-4.4016, -98.5366)
  line L1322 (-4.8287, -97.5056) -> (-4.8398, -97.2233)
  line L1323 (17.9495, -99.6352) -> (17.7654, -99.6132)
  line L1324 (17.1709, -99.2) -> (17.0862, -99.0351)
  line L1325 (-4.6885, -98.0515) -> (-4.7779, -97.7835)
  line L1326 (-0.9202, -96.7281) -> (-0.8607, -97.0043)
  line L1327 (-2.5279, -95.3107) -> (-2.2527, -95.3745)
  line L1328 (-2.2527, -95.3745) -> (-1.9892, -95.4764)
  line L1329 (18.8373, -99.0718) -> (18.7457, -99.233)
  line L1330 (-1.3199, -95.9872) -> (-1.1521, -96.2144)
  line L1331 (17.5891, -99.5559) -> (17.4273, -99.4655)
  line L1332 (17.1856, -98.1487) -> (17.3048, -98.0066)
  line L1333 (17.7914, -97.7522) -> (17.9761, -97.7354)
  line L1334 (18.6246, -99.3734) -> (18.4785, -99.4875)
  line L1335 (17.7654, -99.6132) -> (17.5891, -99.5559)
  line L1336 (18.9194, -98.6854) -> (18.9191, -98.7119)
  line L1337 (17.9761, -97.7354) -> (18.1605, -97.7548)
  line L1338 (17.4493, -97.8905) -> (17.6136, -97.8046)
  line L1339 (-1.5181, -95.7859) -> (-1.3199, -95.9872)
  line L1340 (18.7457, -99.233) -> (18.6246, -99.3734)
  line L1341 (17.4273, -99.4655) -> (17.2861, -99.3453)
  line L1342 (18.9191, -98.7119) -> (18.8958, -98.8959)
  line L1343 (-4.5622, -98.3042) -> (-4.6885, -98.0515)
  line L1344 (18.1344, -99.621) -> (17.9495, -99.6352)
  line L1345 (-3.9908, -98.9224) -> (-4.2099, -98.744)
  line L1346 (17.0402, -98.4879) -> (17.0963, -98.3111)
  line L1347 (18.313, -99.5711) -> (18.1344, -99.621)
  line L1348 (-3.3685, -95.357) -> (-3.0914, -95.3019)
  line L1349 (-4.8398, -97.2233) -> (-4.811, -96.9422)
  line L1350 (3.0404, -97.8062) -> (3.094, -97.9837)
  line L1351 (2.1422, -99.118) -> (1.9581, -99.0961)
  line L1352 (1.7817, -99.0388) -> (1.6199, -98.9483)
  line L1353 (-3.2155, -99.2507) -> (-3.4886, -99.1783)
  line L1354 (3.1121, -98.1682) -> (3.1117, -98.1947)
  line L1355 (-0.8408, -97.2861) -> (-0.8447, -97.4117)
  line L1356 (-2.6525, -99.2772) -> (-2.935, -99.2839)
  line L1357 (1.6199, -98.9483) -> (1.4787, -98.8281)
  line L1358 (-1.6149, -98.8664) -> (-1.8498, -99.0233)
  line L1359 (2.6933, -97.3806) -> (2.8362, -97.4988)
  line L1360 (1.2122, -98.155) -> (1.2328, -97.9707)
  line L1361 (-1.1521, -96.2144) -> (-1.0179, -96.4631)
  line L1362 (2.6711, -98.9703) -> (2.5056, -99.0539)
  line L1363 (-4.32, -95.9401) -> (-4.1156, -95.7451)
  line L1364 (-3.4886, -99.1783) -> (-3.7487, -99.0681)
  line L1365 (-4.1156, -95.7451) -> (-3.8857, -95.5808)
  line L1366 (2.3531, -97.2376) -> (2.5302, -97.2924)
  line L1367 (2.5056, -99.0539) -> (2.327, -99.1038)
  line L1368 (-2.935, -99.2839) -> (-3.2155, -99.2507)
  line L1369 (2.9384, -98.7158) -> (2.8172, -98.8562)
  line L1370 (2.8172, -98.8562) -> (2.6711, -98.9703)
  line L1371 (-3.8857, -95.5808) -> (-3.6351, -95.4506)
  line L1372 (3.1117, -98.1947) -> (3.0885, -98.3787)
  line L1373 (-1.4045, -98.6779) -> (-1.6149, -98.8664)
  line L1374 (-4.811, -96.9422) -> (-4.7429, -96.668)
  line L1375 (-1.2227, -98.4617) -> (-1.4045, -98.6779)
  line L1376 (-3.6351, -95.4506) -> (-3.3685, -95.357)
  line L1377 (1.3635, -98.6828) -> (1.2788, -98.5179)
  line L1378 (-2.8093, -95.2863) -> (-2.5279, -95.3107)
  line L1379 (2.8362, -97.4988) -> (2.9533, -97.6425)
  line L1380 (215.704, -95.5878) -> (215.872, -95.8151)
  line L1381 (216.065, -97.5642) -> (215.951, -97.8226)
  line L1382 (3.0299, -98.5546) -> (2.9384, -98.7158)
  line L1383 (2.5302, -97.2924) -> (2.6933, -97.3806)
  line L1384 (-2.1045, -99.1456) -> (-2.3739, -99.2308)
  line L1385 (-0.959, -97.9636) -> (-1.0732, -98.2219)
  line L1386 (-4.4949, -96.1619) -> (-4.32, -95.9401)
  line L1387 (1.2788, -98.5179) -> (1.2277, -98.3397)
  line L1388 (2.327, -99.1038) -> (2.1422, -99.118)
  line L1389 (1.2277, -98.3397) -> (1.2122, -98.155)
  line L1390 (1.4787, -98.8281) -> (1.3635, -98.6828)
  line L1391 (-4.4016, -98.5366) -> (-4.5622, -98.3042)
  line L1392 (-1.0732, -98.2219) -> (-1.2227, -98.4617)
  line L1393 (3.094, -97.9837) -> (3.1121, -98.1682)
  line L1394 (1.9581, -99.0961) -> (1.7817, -99.0388)
  line L1395 (1.2328, -97.9707) -> (1.2889, -97.794)
  line L1396 (214.496, -94.9113) -> (214.771, -94.9751)
  line L1397 (1.2889, -97.794) -> (1.3782, -97.6315)
  line L1398 (1.8062, -97.2874) -> (1.9841, -97.235)
  line L1399 (215.872, -95.8151) -> (216.006, -96.0637)
  line L1400 (2.9533, -97.6425) -> (3.0404, -97.8062)
  line L1401 (216.179, -97.0123) -> (216.142, -97.2923)
  line L1402 (-0.8823, -97.6917) -> (-0.959, -97.9636)
  line L1403 (-3.7487, -99.0681) -> (-3.9908, -98.9224)
  line L1404 (-0.8607, -97.0043) -> (-0.8408, -97.2861)
  line L1405 (-1.0179, -96.4631) -> (-0.9202, -96.7281)
  line L1406 (-4.7779, -97.7835) -> (-4.8287, -97.5056)
  line L1407 (3.0885, -98.3787) -> (3.0299, -98.5546)
  line L1408 (-2.3739, -99.2308) -> (-2.6525, -99.2772)
  line L1409 (-3.0914, -95.3019) -> (-2.8093, -95.2863)
  line L1410 (317.263, -98.3634) -> (317.317, -98.5409)
  line L1411 (132.995, -99.444) -> (132.979, -99.2592)
  line L1412 (133.573, -98.3917) -> (133.751, -98.3393)
  line L1413 (134.584, -99.9605) -> (134.438, -100.075)
  line L1414 (133.909, -100.222) -> (133.725, -100.2)
  line L1415 (317.317, -98.5409) -> (317.335, -98.7255)
  line L1416 (134.856, -99.483) -> (134.797, -99.6589)
  line L1417 (134.273, -100.158) -> (134.094, -100.208)
  line L1418 (134.438, -100.075) -> (134.273, -100.158)
  line L1419 (317.335, -98.7255) -> (317.335, -98.752)
  line L1420 (134.797, -99.6589) -> (134.705, -99.8201)
  line L1421 (18.7607, -98.1597) -> (18.8478, -98.3234)
  line L1422 (317.253, -99.1119) -> (317.161, -99.2731)
  line L1423 (316.392, -97.7755) -> (316.576, -97.7949)
  line L1424 (315.601, -98.1887) -> (315.72, -98.0467)
  line L1425 (18.5007, -97.8978) -> (18.6435, -98.016)
  line L1426 (315.843, -99.5055) -> (315.702, -99.3854)
  line L1427 (133.387, -100.053) -> (133.246, -99.9324)
  line L1428 (133.056, -98.8983) -> (133.145, -98.7358)
  line L1429 (134.094, -100.208) -> (133.909, -100.222)
  line L1430 (317.161, -99.2731) -> (317.04, -99.4134)
  line L1431 (18.8478, -98.3234) -> (18.9013, -98.5009)
  line L1432 (18.6435, -98.016) -> (18.7607, -98.1597)
  line L1433 (18.9013, -98.5009) -> (18.9194, -98.6854)
  line L1434 (133.046, -99.6222) -> (132.995, -99.444)
  line L1435 (316.729, -99.6112) -> (316.55, -99.661)
  line L1436 (317.04, -99.4134) -> (316.894, -99.5276)
  line L1437 (133.246, -99.9324) -> (133.131, -99.7871)
  line L1438 (316.005, -99.596) -> (315.843, -99.5055)
  line L1439 (317.311, -98.9359) -> (317.253, -99.1119)
  line L1440 (316.894, -99.5276) -> (316.729, -99.6112)
  line L1441 (316.55, -99.661) -> (316.365, -99.6752)
  line L1442 (315.702, -99.3854) -> (315.587, -99.2401)
  line L1443 (316.181, -99.6533) -> (316.005, -99.596)
  line L1444 (315.72, -98.0467) -> (315.865, -97.9305)
  line L1445 (134.705, -99.8201) -> (134.584, -99.9605)
  line L1446 (316.365, -99.6752) -> (316.181, -99.6533)
  line L1447 (315.435, -98.7122) -> (315.456, -98.5279)
  line L1448 (315.865, -97.9305) -> (316.029, -97.8446)
  line L1449 (316.029, -97.8446) -> (316.207, -97.7923)
  line L1450 (316.207, -97.7923) -> (316.392, -97.7755)
  line L1451 (315.451, -98.8969) -> (315.435, -98.7122)
  line L1452 (317.335, -98.752) -> (317.311, -98.9359)
  line L1453 (18.1605, -97.7548) -> (18.3376, -97.8096)
  line L1454 (315.502, -99.0752) -> (315.451, -98.8969)
  line L1455 (315.587, -99.2401) -> (315.502, -99.0752)
  line L1456 (315.456, -98.5279) -> (315.512, -98.3512)
  line L1457 (315.512, -98.3512) -> (315.601, -98.1887)
  line L1458 (18.3376, -97.8096) -> (18.5007, -97.8978)
  line L1459 (-1.7427, -95.6145) -> (-1.5181, -95.7859)
  line L1460 (32.2327, -81.7156) -> (32.2095, -81.8995)
  line L1461 (30.3538, -81.4916) -> (30.4099, -81.3148)
  line L1462 (32.0594, -82.2367) -> (31.9382, -82.377)
  line L1463 (197.308, -79.6214) -> (197.485, -79.6762)
  line L1464 (197.909, -80.0263) -> (197.996, -80.19)
  line L1465 (198.049, -80.3675) -> (198.067, -80.552)
  line L1466 (198.067, -80.552) -> (198.067, -80.5785)
  line L1467 (30.4992, -81.1524) -> (30.6184, -81.0103)
  line L1468 (30.9028, -82.5596) -> (30.7409, -82.4692)
  line L1469 (30.3332, -81.6758) -> (30.3538, -81.4916)
  line L1470 (197.791, -79.8826) -> (197.909, -80.0263)
  line L1471 (31.2897, -80.7391) -> (31.4741, -80.7585)
  line L1472 (31.0791, -82.6169) -> (30.9028, -82.5596)
  line L1473 (197.996, -80.19) -> (198.049, -80.3675)
  line L1474 (31.6266, -82.5748) -> (31.4481, -82.6246)
  line L1475 (30.3998, -82.0388) -> (30.3487, -81.8606)
  line L1476 (140.444, -80.5142) -> (140.586, -80.2699)
  line L1477 (141.712, -79.4649) -> (141.989, -79.4098)
  line L1478 (187.48, -81.4405) -> (187.643, -81.5287)
  line L1479 (140.241, -81.3312) -> (140.27, -81.0502)
  line L1480 (188.044, -82.1317) -> (188.062, -82.3163)
  line L1481 (140.586, -80.2699) -> (140.761, -80.048)
  line L1482 (141.195, -79.6888) -> (141.446, -79.5585)
  line L1483 (141.332, -83.1761) -> (141.09, -83.0304)
  line L1484 (142.428, -83.3852) -> (142.146, -83.3918)
  line L1485 (187.643, -81.5287) -> (187.786, -81.6469)
  line L1486 (141.592, -83.2862) -> (141.332, -83.1761)
  line L1487 (187.903, -81.7905) -> (187.99, -81.9542)
  line L1488 (140.519, -82.4121) -> (140.392, -82.1594)
  line L1489 (187.303, -81.3857) -> (187.48, -81.4405)
  line L1490 (187.99, -81.9542) -> (188.044, -82.1317)
  line L1491 (141.865, -83.3586) -> (141.592, -83.2862)
  line L1492 (140.252, -81.6135) -> (140.241, -81.3312)
  line L1493 (140.303, -81.8914) -> (140.252, -81.6135)
  line L1494 (142.146, -83.3918) -> (141.865, -83.3586)
  line L1495 (140.679, -82.6445) -> (140.519, -82.4121)
  line L1496 (140.392, -82.1594) -> (140.303, -81.8914)
  line L1497 (140.761, -80.048) -> (140.965, -79.853)
  line L1498 (141.989, -79.4098) -> (142.271, -79.3943)
  line L1499 (187.277, -83.2518) -> (187.092, -83.266)
  line L1500 (187.98, -82.7027) -> (187.888, -82.8639)
  line L1501 (186.447, -81.6375) -> (186.591, -81.5213)
  line L1502 (188.038, -82.5267) -> (187.98, -82.7027)
  line L1503 (187.767, -83.0042) -> (187.621, -83.1184)
  line L1504 (147.434, -81.3456) -> (147.611, -81.4004)
  line L1505 (186.908, -83.2441) -> (186.731, -83.1868)
  line L1506 (186.428, -82.9762) -> (186.313, -82.8309)
  line L1507 (186.239, -81.942) -> (186.328, -81.7795)
  line L1508 (141.446, -79.5585) -> (141.712, -79.4649)
  line L1509 (186.328, -81.7795) -> (186.447, -81.6375)
  line L1510 (186.57, -83.0963) -> (186.428, -82.9762)
  line L1511 (186.182, -82.1187) -> (186.239, -81.942)
  line L1512 (148.034, -81.7505) -> (148.121, -81.9142)
  line L1513 (188.061, -82.3428) -> (188.038, -82.5267)
  line L1514 (186.591, -81.5213) -> (186.756, -81.4354)
  line L1515 (148.121, -81.9142) -> (148.175, -82.0917)
  line L1516 (188.062, -82.3163) -> (188.061, -82.3428)
  line L1517 (186.162, -82.303) -> (186.182, -82.1187)
  line L1518 (187.118, -81.3663) -> (187.303, -81.3857)
  line L1519 (147.774, -81.4886) -> (147.917, -81.6068)
  line L1520 (147.917, -81.6068) -> (148.034, -81.7505)
  line L1521 (187.455, -83.202) -> (187.277, -83.2518)
  line L1522 (187.888, -82.8639) -> (187.767, -83.0042)
  line L1523 (147.611, -81.4004) -> (147.774, -81.4886)
  line L1524 (187.621, -83.1184) -> (187.455, -83.202)
  line L1525 (187.092, -83.266) -> (186.908, -83.2441)
  line L1526 (186.313, -82.8309) -> (186.228, -82.666)
  line L1527 (186.934, -81.3831) -> (187.118, -81.3663)
  line L1528 (186.177, -82.4877) -> (186.162, -82.303)
  line L1529 (146.293, -82.2629) -> (146.314, -82.0787)
  line L1530 (148.111, -82.6626) -> (148.019, -82.8238)
  line L1531 (186.228, -82.666) -> (186.177, -82.4877)
  line L1532 (147.408, -83.2118) -> (147.223, -83.226)
  line L1533 (146.36, -82.6259) -> (146.308, -82.4477)
  line L1534 (148.169, -82.4867) -> (148.111, -82.6626)
  line L1535 (146.444, -82.7908) -> (146.36, -82.6259)
  line L1536 (146.308, -82.4477) -> (146.293, -82.2629)
  line L1537 (148.192, -82.3027) -> (148.169, -82.4867)
  line L1538 (147.065, -81.343) -> (147.249, -81.3262)
  line L1539 (147.249, -81.3262) -> (147.434, -81.3456)
  line L1540 (308.926, -79.0373) -> (309.172, -79.1754)
  line L1541 (146.701, -83.0563) -> (146.559, -82.9361)
  line L1542 (309.172, -79.1754) -> (309.397, -79.3468)
  line L1543 (146.862, -83.1467) -> (146.701, -83.0563)
  line L1544 (186.756, -81.4354) -> (186.934, -81.3831)
  line L1545 (308.662, -78.9354) -> (308.926, -79.0373)
  line L1546 (147.752, -83.0783) -> (147.586, -83.1619)
  line L1547 (147.039, -83.204) -> (146.862, -83.1467)
  line L1548 (146.559, -82.9361) -> (146.444, -82.7908)
  line L1549 (147.586, -83.1619) -> (147.408, -83.2118)
  line L1550 (146.459, -81.7395) -> (146.578, -81.5974)
  line L1551 (146.578, -81.5974) -> (146.723, -81.4813)
  line L1552 (148.175, -82.0917) -> (148.193, -82.2762)
  line L1553 (148.019, -82.8238) -> (147.898, -82.9641)
  line L1554 (309.397, -79.3468) -> (309.595, -79.5481)
  line L1555 (147.223, -83.226) -> (147.039, -83.204)
  line L1556 (186.731, -83.1868) -> (186.57, -83.0963)
  line L1557 (148.193, -82.2762) -> (148.192, -82.3027)
  line L1558 (147.898, -82.9641) -> (147.752, -83.0783)
  line L1559 (308.81, -82.7066) -> (308.541, -82.7917)
  line L1560 (307.426, -82.7392) -> (307.166, -82.629)
  line L1561 (306.924, -82.4833) -> (306.705, -82.3049)
  line L1562 (310.054, -80.5652) -> (310.074, -80.847)
  line L1563 (306.353, -81.8651) -> (306.226, -81.6124)
  line L1564 (307.166, -82.629) -> (306.924, -82.4833)
  line L1565 (306.137, -81.3444) -> (306.086, -81.0665)
  line L1566 (309.51, -82.2388) -> (309.3, -82.4273)
  line L1567 (306.086, -81.0665) -> (306.075, -80.7842)
  line L1568 (308.541, -82.7917) -> (308.262, -82.8381)
  line L1569 (308.262, -82.8381) -> (307.98, -82.8448)
  line L1570 (309.842, -81.7829) -> (309.692, -82.0226)
  line L1571 (309.595, -79.5481) -> (309.763, -79.7753)
  line L1572 (306.104, -80.5031) -> (306.172, -80.229)
  line L1573 (309.692, -82.0226) -> (309.51, -82.2388)
  line L1574 (306.075, -80.7842) -> (306.104, -80.5031)
  line L1575 (307.699, -82.8116) -> (307.426, -82.7392)
  line L1576 (306.705, -82.3049) -> (306.513, -82.0975)
  line L1577 (309.065, -82.5843) -> (308.81, -82.7066)
  line L1578 (306.226, -81.6124) -> (306.137, -81.3444)
  line L1579 (309.995, -80.289) -> (310.054, -80.5652)
  line L1580 (309.763, -79.7753) -> (309.897, -80.024)
  line L1581 (146.887, -81.3954) -> (147.065, -81.343)
  line L1582 (146.314, -82.0787) -> (146.37, -81.9019)
  line L1583 (146.723, -81.4813) -> (146.887, -81.3954)
  line L1584 (308.387, -78.8716) -> (308.662, -78.9354)
  line L1585 (146.37, -81.9019) -> (146.459, -81.7395)
  line L1586 (25.3723, -82.5889) -> (25.1303, -82.4432)
  line L1587 (303.44, -80.8534) -> (303.603, -80.9415)
  line L1588 (26.3117, -78.8072) -> (26.5931, -78.8316)
  line L1589 (28.2763, -80.9325) -> (28.2387, -81.2125)
  line L1590 (24.9112, -82.2649) -> (24.7194, -82.0574)
  line L1591 (307.28, -79.0115) -> (307.546, -78.9179)
  line L1592 (24.4842, -79.9271) -> (24.6261, -79.6828)
  line L1593 (26.5931, -78.8316) -> (26.8683, -78.8954)
  line L1594 (304.021, -81.7291) -> (304.021, -81.7557)
  line L1595 (306.42, -79.7228) -> (306.595, -79.501)
  line L1596 (307.824, -78.8628) -> (308.106, -78.8473)
  line L1597 (25.7525, -78.8778) -> (26.0296, -78.8227)
  line L1598 (24.7194, -82.0574) -> (24.5588, -81.825)
  line L1599 (27.6029, -79.3067) -> (27.8011, -79.508)
  line L1600 (306.595, -79.501) -> (306.799, -79.306)
  line L1601 (25.0054, -79.2659) -> (25.2353, -79.1017)
  line L1602 (303.863, -81.2034) -> (303.95, -81.3671)
  line L1603 (306.513, -82.0975) -> (306.353, -81.8651)
  line L1604 (26.4685, -82.7981) -> (26.186, -82.8047)
  line L1605 (310.07, -80.9726) -> (310.033, -81.2526)
  line L1606 (27.5061, -82.3872) -> (27.2712, -82.5442)
  line L1607 (26.7472, -82.7517) -> (26.4685, -82.7981)
  line L1608 (27.1318, -78.9973) -> (27.3783, -79.1353)
  line L1609 (303.998, -81.9396) -> (303.939, -82.1155)
  line L1610 (27.2712, -82.5442) -> (27.0165, -82.6665)
  line L1611 (28.2387, -81.2125) -> (28.162, -81.4844)
  line L1612 (28.1031, -79.9839) -> (28.2008, -80.249)
  line L1613 (27.9689, -79.7353) -> (28.1031, -79.9839)
  line L1614 (25.1303, -82.4432) -> (24.9112, -82.2649)
  line L1615 (303.603, -80.9415) -> (303.746, -81.0597)
  line L1616 (26.0296, -78.8227) -> (26.3117, -78.8072)
  line L1617 (306.172, -80.229) -> (306.278, -79.9671)
  line L1618 (28.2008, -80.249) -> (28.2603, -80.5251)
  line L1619 (25.9055, -82.7715) -> (25.6324, -82.6991)
  line L1620 (26.186, -82.8047) -> (25.9055, -82.7715)
  line L1621 (24.6261, -79.6828) -> (24.801, -79.4609)
  line L1622 (24.31, -80.4631) -> (24.3781, -80.1889)
  line L1623 (307.029, -79.1417) -> (307.28, -79.0115)
  line L1624 (309.897, -80.024) -> (309.995, -80.289)
  line L1625 (27.3783, -79.1353) -> (27.6029, -79.3067)
  line L1626 (307.546, -78.9179) -> (307.824, -78.8628)
  line L1627 (24.3431, -81.3043) -> (24.2923, -81.0264)
  line L1628 (28.2803, -80.8069) -> (28.2763, -80.9325)
  line L1629 (306.799, -79.306) -> (307.029, -79.1417)
  line L1630 (27.0165, -82.6665) -> (26.7472, -82.7517)
  line L1631 (28.2603, -80.5251) -> (28.2803, -80.8069)
  line L1632 (27.8983, -81.9825) -> (27.7165, -82.1988)
  line L1633 (27.8011, -79.508) -> (27.9689, -79.7353)
  line L1634 (303.939, -82.1155) -> (303.848, -82.2767)
  line L1635 (310.033, -81.2526) -> (309.956, -81.5245)
  line L1636 (307.98, -82.8448) -> (307.699, -82.8116)
  line L1637 (309.3, -82.4273) -> (309.065, -82.5843)
  line L1638 (26.8683, -78.8954) -> (27.1318, -78.9973)
  line L1639 (306.278, -79.9671) -> (306.42, -79.7228)
  line L1640 (310.074, -80.847) -> (310.07, -80.9726)
  line L1641 (28.0478, -81.7428) -> (27.8983, -81.9825)
  line L1642 (25.486, -78.9714) -> (25.7525, -78.8778)
  line L1643 (28.162, -81.4844) -> (28.0478, -81.7428)
  line L1644 (308.106, -78.8473) -> (308.387, -78.8716)
  line L1645 (309.956, -81.5245) -> (309.842, -81.7829)
  line L1646 (27.7165, -82.1988) -> (27.5061, -82.3872)
  line L1647 (24.4325, -81.5723) -> (24.3431, -81.3043)
  line L1648 (32.2095, -81.8995) -> (32.151, -82.0755)
  line L1649 (302.551, -80.9342) -> (302.716, -80.8483)
  line L1650 (303.078, -80.7792) -> (303.262, -80.7985)
  line L1651 (24.2923, -81.0264) -> (24.2812, -80.7441)
  line L1652 (304.021, -81.7557) -> (303.998, -81.9396)
  line L1653 (302.867, -82.657) -> (302.691, -82.5997)
  line L1654 (303.415, -82.6148) -> (303.236, -82.6647)
  line L1655 (24.3781, -80.1889) -> (24.4842, -79.9271)
  line L1656 (303.727, -82.4171) -> (303.58, -82.5312)
  line L1657 (302.122, -81.7159) -> (302.142, -81.5316)
  line L1658 (302.288, -81.1924) -> (302.407, -81.0504)
  line L1659 (31.9572, -81.0197) -> (32.0744, -81.1633)
  line L1660 (302.893, -80.796) -> (303.078, -80.7792)
  line L1661 (32.2331, -81.6891) -> (32.2327, -81.7156)
  line L1662 (25.6324, -82.6991) -> (25.3723, -82.5889)
  line L1663 (302.691, -82.5997) -> (302.529, -82.5092)
  line L1664 (302.529, -82.5092) -> (302.388, -82.3891)
  line L1665 (32.215, -81.5045) -> (32.2331, -81.6891)
  line L1666 (303.58, -82.5312) -> (303.415, -82.6148)
  line L1667 (303.848, -82.2767) -> (303.727, -82.4171)